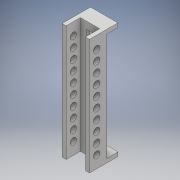
# Autodesk Inventor part: slider-rail-adapter
Saved by Autodesk Inventor 2018 (Build 220112000, 112)
## iProperties
Created: 2025-03-03
Part Number: slider-rail-adapter
Material: Generic
Document SubType Name: Modeling
Designer: neo
Density: 1 g/cm^3
Appearance: Default
Author: neo
Autodesk Inventor part; units mm, degrees
ref_plane "YZ Plane" through (0, 0, 0) normal (1, 0, 0) x (0, 1, 0)
ref_plane "XZ Plane" through (0, 0, 0) normal (0, 1, 0) x (-1, 0, 0)
ref_plane "XY Plane" through (0, 0, 0) normal (0, 0, 1) x (1, 0, 0)
sketch "Sketch1" plane through (0, 0, 0) normal (0, 1, 0) x (-1, 0, 0)
  line L0 (2.7098, 27.525) -> (-10.7902, 27.525)
  line L1 (-10.7902, 27.525) -> (-10.7902, -29.475)
  line L2 (-10.7902, -29.475) -> (2.7098, -29.475)
  line L3 (2.7098, -29.475) -> (2.7098, 27.525)
  line L4 (-4.0402, 27.525) -> (-4.0402, -29.475)
  line L5 (0.7098, 27.525) -> (0.7098, -29.475)
  line L6 (-8.7902, 27.525) -> (-8.7902, -29.475)
  line L7 (-8.7902, 27.525) -> (-10.7902, 27.525)
  line L8 (-10.7902, 27.525) -> (-10.7902, -29.475)
  line L9 (-10.7902, -29.475) -> (-8.7902, -29.475)
  line L10 (-8.7902, -29.475) -> (-8.7902, 27.525)
  line L11 (2.7098, -29.475) -> (0.7098, -29.475)
  line L12 (0.7098, -29.475) -> (0.7098, 27.525)
  line L13 (0.7098, 27.525) -> (2.7098, 27.525)
  line L14 (2.7098, 27.525) -> (2.7098, -29.475)
  dimension "d31" = 57
  dimension "d33" = 2
  dimension "d34" = 9.5
  constraints: 30 end point, 6 parallel, 4 perpendicular, 3 horizontal, 2 midpoint, 2 point on line, 2 symmetric about line
  measures "d31" distance of L2.end L0.start
  measures "d33" distance between parallel lines of L5 L3
  measures "d34" distance between parallel lines of L6 L5
extrude "Extrusion6" add sketch "Sketch1" along normal blind 5 contours L3 L2 L5 L0 | L6 L2 L1 L0
extrude "Extrusion7" add sketch "Sketch1" against normal blind 2
sketch "Sketch4" plane through (-2.7098, 5, -29.475) normal (-1, 0, 0) x (0, 0, 1)
  line L0 (57, -7) -> (57, 0) construction
  line L1 (0, 0) -> (57, 0) construction
  line L2 (0, -7) -> (0, 0) construction
  line L3 (57, -7) -> (0, -7) construction
  line L4 (55, 0) -> (2, 0)
  line L5 (2, 0) -> (2, -5.5)
  line L6 (2, -5.5) -> (55, -5.5)
  line L7 (55, -5.5) -> (55, 0)
  point P0 (29.475, -5)
  dimension "d39" = 2
  dimension "d40" = 2
  dimension "d41" = 1.5
  constraints: 8 end point, 2 parallel, 1 horizontal, 1 perpendicular, 1 point on line
  measures "d39" distance between parallel lines of L0 L7
  measures "d40" distance between parallel lines of L2 L5
  measures "d41" distance between parallel lines of L3 L6
extrude "Extrusion8" cut sketch "Sketch4" against normal up to surface (13.5 mm away)
sketch "Sketch5" plane through (8.7902, 0, 27.525) normal (-1, 0, 0) x (0, 0, 1)
  line L0 (-2, 5) -> (-2, 0) projected
  line L1 (-2, 0) -> (0, 0) projected
  line L2 (0, 0) -> (0, 5) projected
  line L3 (-2, 5) -> (0, 5) projected
  line L4 (-55, 0) -> (-55, 5) projected
  line L5 (-57, 5) -> (-55, 5) projected
  line L6 (-57, 0) -> (-57, 5) projected
  line L7 (-57, 0) -> (-55, 0) projected
  point P0 (-27.525, 0)
extrude "Extrusion9" add sketch "Sketch5" along normal through all both and the other way through all
sketch "Sketch6" plane through (0, -2, 0) normal (0, -1, 0) x (1, 0, 0)
  line L0 (10.7902, 27.525) -> (-2.7098, 27.525) construction
  line L1 (-2.7098, 27.525) -> (-2.7098, -29.475) construction
  line L2 (-2.7098, -29.475) -> (10.7902, -29.475) construction
  line L3 (10.7902, -29.475) -> (10.7902, 27.525) construction
  line L4 (4.0402, 32.9205) -> (4.0402, -29.475)
  line L5 (5.6402, 24.1195) -> (2.4402, 24.1195)
  line L6 (2.4402, 24.1195) -> (2.4402, -25.8805)
  line L7 (2.4402, -25.8805) -> (5.6402, -25.8805)
  line L8 (5.6402, -25.8805) -> (5.6402, 24.1195)
  point P0 (0, 0)
  dimension "d46" = 50
  dimension "d47" = 3.2
  constraints: 10 end point, 2 parallel, 1 horizontal, 1 midpoint, 1 perpendicular, 1 other
  measures "d46" distance between parallel lines of L7 L5
  measures "d47" distance between parallel lines of L6 L8
extrude "Extrusion10" cut sketch "Sketch6" against normal through all
sketch "Sketch7" plane through (0, -2, 0) normal (0, -1, 0) x (1, 0, 0)
  line L0 (2.4402, -25.8805) -> (2.4402, 24.1195) construction
  line L1 (2.4402, 24.1195) -> (5.6402, 24.1195) construction
  line L2 (5.6402, 24.1195) -> (5.6402, -25.8805) construction
  line L3 (5.6402, -25.8805) -> (2.4402, -25.8805) construction
  line L4 (10.7902, 27.525) -> (-2.7098, 27.525) construction
  line L5 (-2.7098, 27.525) -> (-2.7098, -29.475) construction
  line L6 (-2.7098, -29.475) -> (10.7902, -29.475) construction
  line L7 (10.7902, -29.475) -> (10.7902, 27.525) construction
  line L8 (-2.7098, 27.525) -> (-0.7098, 27.525)
  line L9 (-0.7098, 27.525) -> (-0.7098, -29.475)
  line L10 (-0.7098, -29.475) -> (-2.7098, -29.475)
  line L11 (-2.7098, -29.475) -> (-2.7098, 27.525)
  line L12 (10.7902, 27.525) -> (8.7902, 27.525)
  line L13 (8.7902, 27.525) -> (8.7902, -29.475)
  line L14 (8.7902, -29.475) -> (10.7902, -29.475)
  line L15 (10.7902, -29.475) -> (10.7902, 27.525)
  line L16 (-2.7098, -29.475) -> (10.7902, -29.475) projected
  point P0 (0, 0)
  dimension "d50" = 2
  dimension "d51" = 2
  constraints: 16 end point, 4 parallel, 2 horizontal, 2 perpendicular, 2 point on line
  measures "d50" distance between parallel lines of L13 L7
  measures "d51" distance between parallel lines of L5 L9
extrude "Extrusion11" add sketch "Sketch7" along normal blind 7
sketch "Sketch8" plane through (-2.7098, -0.5, 25.525) normal (-1, 0, 0) x (0, 0, 1)
  line L0 (2, -8.5) -> (2, 5.5) construction
  line L1 (0, 5.5) -> (2, 5.5) construction
  line L2 (0, 5.5) -> (0, 0) construction
  line L3 (0, 0) -> (-53, 0) construction
  line L4 (-53, 0) -> (-53, 5.5) construction
  line L5 (-55, 5.5) -> (-53, 5.5) construction
  line L6 (-55, -8.5) -> (-55, 5.5) construction
  line L7 (2, -8.5) -> (-55, -8.5) construction
  line L8 (-55, -8.5) -> (-55, 5.5) construction
  line L9 (2, -8.5) -> (-55, -8.5) construction
  line L10 (-55, -8.5) -> (-55, 0) construction
  line L11 (-55, 0) -> (2, 0) construction
  line L12 (2, 0) -> (2, -8.5) construction
  circle A0 centre (-4, -5) radius 1.6
  point P0 (-25.525, 0.5)
  dimension "d54" = 3.2
  dimension "d55" = 5
  dimension "d56" = 6
  constraints: 8 end point, 2 parallel, 1 centre point, 1 horizontal, 1 perpendicular, 1 point on line
  measures "d54" diameter of A0
  measures "d55" distance from line of L3 A0.centre
  measures "d56" distance from line of L0 A0.centre
extrude "Extrusion12" cut sketch "Sketch8" against normal through all
pattern_linear "Rectangular Pattern3" count 10 spacing 5 along (0, 0, -1) of "Extrusion12"
body "Solid2"
